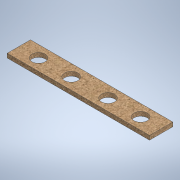
# Autodesk Inventor part: Estructura Anillos
Saved by Autodesk Inventor 2020 (Build 240168000, 168)
## iProperties
Created: 2021-09-30
Part Number: Estructura Anillos
Material: MDF Medium Density Fiberboard
Document SubType Name: Modeling
Designer: Carlos
Density: 0.8 g/cm^3
Appearance: Cardboard - Corrugated
Author: Carlos
Autodesk Inventor part; units mm, degrees
ref_plane "YZ Plane" through (0, 0, 0) normal (1, 0, 0) x (0, 1, 0)
ref_plane "XZ Plane" through (0, 0, 0) normal (0, 1, 0) x (-1, 0, 0)
ref_plane "XY Plane" through (0, 0, 0) normal (0, 0, 1) x (1, 0, 0)
sketch "Sketch1" plane through (0, 0, 0) normal (0, 1, 0) x (-1, 0, 0)
  line L0 (0, 0) -> (0, -14)
  line L1 (0, -14) -> (85.598, -14)
  line L2 (85.598, -14) -> (85.598, 0)
  line L3 (85.598, 0) -> (0, 0)
  dimension "d0" = 14
  dimension "d1" = 85.598
  constraints: 8 end point, 3 perpendicular, 1 vertical
  measures "d0" distance of L0.start L0.end
  measures "d1" distance of L0.end L1.end
extrude "Extrusion1" add sketch "Sketch1" along normal blind 2.5
sketch "Sketch2" plane through (0, 2.5, 0) normal (0, 1, 0) x (1, 0, 0)
  line L0 (0, 0) -> (0, 14) projected
  line L1 (0, 14) -> (-85.598, 14) projected
  line L2 (-85.598, 0) -> (0, 0) projected
  circle A0 centre (-12.3165, 7) radius 4
  circle A1 centre (-31.949, 7) radius 4
  line L3 (0, 0) -> (-85.598, 0)
  line L4 (0, 24) -> (-2.5, 24)
  line L5 (-2.5, 24) -> (-41.766, 24)
  line L6 (-41.766, 24) -> (-44.266, 24)
  line L7 (-44.266, 24) -> (-54.083, 24)
  line L8 (-44.266, 24) -> (-83.532, 24)
  line L9 (-83.532, 24) -> (-73.715, 24)
  line L10 (-73.715, 24) -> (-73.715, -12)
  line L11 (-44.266, 24) -> (-44.266, -7)
  line L12 (-54.083, 24) -> (-54.083, -7)
  circle A2 centre (-54.083, 7) radius 4
  circle A3 centre (-73.715, 7) radius 4
  line L13 (-73.715, 7) -> (-12.3165, 7)
  dimension "d15" = 8
  dimension "d17" = 2.5
  dimension "d18" = 39.266
  dimension "d19" = 9.8165
  dimension "d20" = 9.817
  dimension "d21" = 2.5
  dimension "d22" = 9.817
  dimension "d23" = 39.266
  dimension "d24" = 9.817
  dimension "d25" = 8
  dimension "d27" = 8
  constraints: 22 end point, 6 point on line, 4 centre point, 3 horizontal, 2 perpendicular, 1 collinear, 1 vertical
  measures "d15" diameter of A1
  measures "d17" distance of L4.start L4.end
  measures "d18" distance of L4.end L5.end
  measures "d19" horizontal distance of L4.end L13.end
  measures "d20" horizontal distance of A1.centre L5.end
  measures "d21" distance of L5.end L6.end
  measures "d22" distance of L6.end L7.end
  measures "d23" distance of L6.end L8.end
  measures "d24" distance of L8.end L9.end
  measures "d25" diameter of A2
  measures "d27" diameter of A3
extrude "Extrusion2" cut sketch "Sketch2" against normal blind 2.5 contours A0 | A1 L13 | L13 A1 | A2 L13 L12 | L12 L13 A2 | L13 L12 A2 | L12 L13 A2 | A3 L10 | L10 L13 A3 | A3 L13 L10
body "Solid1"
